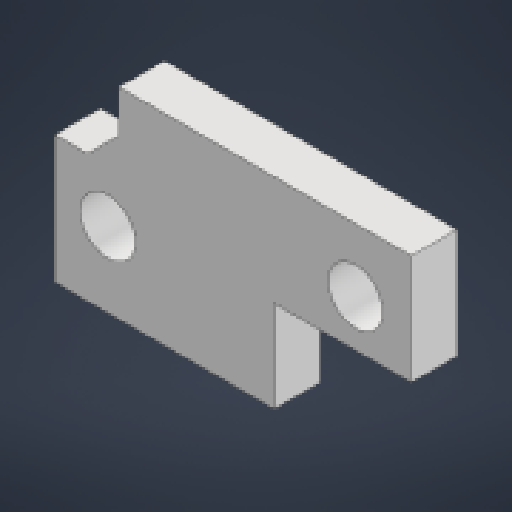
# Autodesk Inventor part: 阻挡X轴
Saved by Autodesk Inventor 2025 (Build 290162000, 162)
## iProperties
Created: 2025-12-13
Part Number: 阻挡X轴
Material: 常规
Document SubType Name: Modeling
Designer: XH
Density: 1 g/cm^3
Appearance: 默认
Author: XH
Autodesk Inventor part; units mm, degrees
ref_plane "YZ Plane" through (0, 0, 0) normal (1, 0, 0) x (0, 1, 0)
ref_plane "XZ Plane" through (0, 0, 0) normal (0, 1, 0) x (-1, 0, 0)
ref_plane "XY Plane" through (0, 0, 0) normal (0, 0, 1) x (1, 0, 0)
sketch "草图1" plane through (0, 0, 0) normal (0, 0, 1) x (1, 0, 0)
  line L0 (3.3485, 1.7155) -> (3.3485, -8.2845) projected
  line L1 (3.3485, -8.2845) -> (-18.6515, -8.2845) projected
  line L2 (-18.6515, -8.2845) -> (-18.6515, 3.7155) projected
  line L3 (-18.6515, 3.7155) -> (-15.6515, 3.7155) projected
  line L4 (-11.6515, 7.7155) -> (-15.6515, 3.7155) projected
  line L5 (-11.6515, 11.7155) -> (-11.6515, 7.7155) projected
  line L6 (18.3485, 11.7155) -> (-11.6515, 11.7155) projected
  line L7 (18.3485, 1.7155) -> (18.3485, 11.7155) projected
  line L8 (18.3485, 1.7155) -> (3.3485, 1.7155) projected
  circle A0 centre (13.2421, 5.8327) radius 3 projected
  circle A1 centre (-13.8563, -1.088) radius 3 projected
  line L9 (-12.6515, 12.7155) -> (-12.6515, 8.1297)
  line L10 (-12.6515, 8.1297) -> (-16.0657, 4.7155)
  line L11 (-16.0657, 4.7155) -> (-19.6515, 4.7155)
  line L12 (-19.6515, 4.7155) -> (-19.6515, -9.2845)
  line L13 (-19.6515, -9.2845) -> (4.3485, -9.2845)
  line L14 (4.3485, -9.2845) -> (4.3485, 0.7155)
  line L15 (4.3485, 0.7155) -> (19.3485, 0.7155)
  line L16 (19.3485, 0.7155) -> (19.3485, 12.7155)
  line L17 (19.3485, 12.7155) -> (-12.6515, 12.7155)
  dimension "d2" = 1
  constraints: 18 end point, 8 other
  measures "d2" distance between parallel lines of L6 L17
extrude "拉伸1" add sketch "草图1" along normal blind 5 contours L0 L1 L2 L3 L4 L5 L6 L7 L8 | L17 L16 L15 L14 L13 L12 L11 L10 L9
